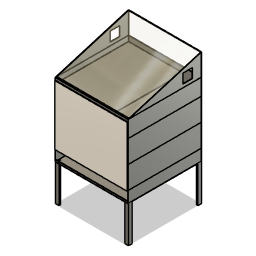
Solar Dryer Assembly v2 (Autodesk Fusion 360 archive; units mm, degrees)
design "Chamber Solar Dryer"
Autodesk Fusion 360 part; units mm, degrees
sketch "Sketch1" plane through (0, 0, 0) normal (0, 1, 0) x (1, 0, 0)
  line L0 (1000, 0) -> (1000, 1000)
  line L1 (1000, 1000) -> (0, 1000)
  line L2 (0, 1000) -> (0, 0)
  line L3 (996, 4) -> (996, 996)
  line L4 (996, 996) -> (4, 996)
  line L5 (4, 996) -> (4, 4)
  line L6 (996, 4) -> (996, 0)
  line L7 (996, 0) -> (1000, 0)
  line L8 (4, 4) -> (4, 0)
  line L9 (4, 0) -> (0, 0)
  dimension "d1" = 1000
  dimension "d2" = 1000
  dimension "d3" = 992
  dimension "d4" = 992
  constraint vertical L0
  constraint horizontal L1
  constraint vertical L2
  constraint coincident L2.end L9.end
  constraint vertical L3
  constraint horizontal L4
  constraint vertical L5
  constraint parallel L0 L6
  constraint perpendicular L0 L7
  constraint perpendicular L7 L8
  constraint perpendicular L2 L9
  measures "d1" distance of L2.end L0.start
  measures "d2" distance of L2.end L1.end
  measures "d3" distance of L5.end L3.start
  measures "d4" distance of L5.end L4.end
extrude "Extrude1" add sketch "Sketch1" along normal blind 1000 makes body 1
ref_plane "WorkPlane1" through (500, 500, -996) normal (0, 0, 1) x (1, 0, 0)
sketch "Sketch2" plane through (0, 0, -996) normal (0, 0, 1) x (1, 0, 0)
  line L0 (4, 0) -> (996, 0)
  line L1 (996, 0) -> (996, 4)
  line L2 (996, 4) -> (4, 4)
  line L3 (4, 4) -> (4, 0)
  dimension "d8" = 992
  dimension "d9" = 4
  constraint horizontal L0
  constraint vertical L1
  constraint horizontal L2
  constraint vertical L3
  measures "d8" distance of L0.start L0.end
  measures "d9" distance of L0.start L2.end
extrude "Extrude2" add sketch "Sketch2" along normal blind 996 bodies 1
ref_plane "WorkPlane2" through (500, 502, -996) normal (0, 0, 1) x (1, 0, 0)
sketch "Sketch3" plane through (0, 0, -996) normal (0, 0, 1) x (1, 0, 0)
  line L0 (4, 312) -> (4, 308)
  line L1 (996, 154) -> (246, 154)
  line L2 (246, 154) -> (246, 158)
  line L3 (246, 158) -> (996, 158)
  line L4 (996, 158) -> (996, 154)
  line L5 (754, 308) -> (754, 312)
  line L6 (754, 312) -> (4, 312)
  line L7 (246, 466) -> (996, 466)
  line L8 (246, 462) -> (246, 466)
  line L9 (996, 462) -> (246, 462)
  line L10 (4, 312) -> (4, 308)
  line L11 (4, 308) -> (754, 308)
  line L12 (996, 466) -> (996, 462)
  line L13 (754, 620) -> (4, 620)
  line L14 (996, 774) -> (996, 770)
  line L15 (246, 774) -> (996, 774)
  line L16 (4, 620) -> (4, 616)
  line L17 (4, 620) -> (4, 616)
  line L18 (996, 770) -> (246, 770)
  line L19 (4, 616) -> (754, 616)
  line L20 (754, 616) -> (754, 620)
  line L21 (246, 770) -> (246, 774)
  line L22 (754, 928) -> (4, 928)
  line L23 (754, 924) -> (754, 928)
  line L24 (4, 924) -> (754, 924)
  line L25 (4, 928) -> (4, 924)
  line L26 (4, 928) -> (4, 924)
  dimension "d14" = 4
  dimension "d15" = 750
  dimension "d16" = 4
  dimension "d17" = 750
  dimension "d18" = 4
  dimension "d19" = 750
  dimension "d20" = 4
  dimension "d21" = 750
  dimension "d22" = 4
  dimension "d24" = 4
  dimension "d25" = 750
  dimension "d26" = 4
  dimension "d27" = 750
  dimension "d28" = 4
  dimension "d30" = 4
  constraint vertical L0
  constraint horizontal L1
  constraint vertical L2
  constraint horizontal L3
  constraint vertical L4
  constraint horizontal L11
  constraint vertical L5
  constraint horizontal L6
  constraint vertical L10
  constraint horizontal L9
  constraint vertical L8
  constraint horizontal L7
  constraint vertical L12
  constraint horizontal L19
  constraint vertical L20
  constraint horizontal L13
  constraint vertical L17
  constraint vertical L16
  constraint horizontal L18
  constraint vertical L21
  constraint horizontal L15
  constraint vertical L14
  constraint horizontal L24
  constraint vertical L23
  constraint horizontal L22
  constraint vertical L26
  constraint vertical L25
  measures "d14" distance of L0.end L0.start
  measures "d15" distance of L1.start L1.end
  measures "d16" distance of L1.start L3.end
  measures "d17" distance of L0.end L5.start
  measures "d18" distance of L0.end L0.start
  measures "d19" distance of L9.start L8.start
  measures "d20" distance of L9.start L7.end
  measures "d21" distance of L16.end L19.end
  measures "d22" distance of L16.end L13.end
  measures "d24" distance of L13.end L16.end
  measures "d25" distance of L18.end L14.end
  measures "d26" distance of L14.end L14.start
  measures "d27" distance of L24.start L23.start
  measures "d28" distance of L24.start L22.end
  measures "d30" distance of L22.end L24.start
extrude "Extrude3" add sketch "Sketch3" along normal blind 992 separate body makes body 2 at (496, 466, -665.3333) makes body 3 at (746, 770, -665.3333) makes body 4 at (504, 312, -665.3333) makes body 5 at (254, 616, -665.3333) makes body 6 at (254, 924, -665.3333) makes body 7 at (746, 154, -665.3333)
ref_plane "WorkPlane3" through (4, 502, -498) normal (1, 0, 0) x (0, 0, -1)
sketch "Sketch4" plane through (4, 0, 0) normal (1, 0, 0) x (0, 0, -1)
  line L0 (1000, 1000) -> (1000, 1300)
  line L1 (1000, 1300) -> (0, 1000)
  line L2 (1000, 1000) -> (996, 1000)
  line L3 (0, 1000) -> (4, 1000)
  line L4 (996, 1000) -> (996, 1293)
  line L5 (996, 1293) -> (996, 1294)
  line L6 (996, 1294) -> (15.9999, 1000)
  line L7 (15.9999, 1000) -> (4, 1000)
  dimension "d34" = 300
  dimension "d35" = 4
  dimension "d36" = 4
  constraint vertical L0
  constraint perpendicular L0 L2
  constraint horizontal L3
  constraint perpendicular L2 L4
  constraint parallel L4 L5
  constraint parallel L1 L6
  constraint parallel L3 L7
  measures "d34" distance of L0.start L0.end
  measures "d35" distance of L0.start L2.end
  measures "d36" distance of L1.end L3.end
extrude "Extrude4" add sketch "Sketch4" along normal blind 992 separate body makes body 8
ref_plane "WorkPlane4" through (379, 926, -4) normal (0, 0, 1) x (1, 0, 0)
sketch "Sketch5" plane through (0, 0, -4) normal (0, 0, 1) x (1, 0, 0)
  line L0 (4, 305) -> (4, 315)
  line L1 (996, 161) -> (246, 161)
  line L2 (246, 161) -> (246, 151)
  line L3 (246, 151) -> (996, 151)
  line L4 (996, 151) -> (996, 161)
  line L5 (996, 767) -> (996, 777)
  line L6 (246, 767) -> (996, 767)
  line L7 (996, 777) -> (246, 777)
  line L8 (246, 777) -> (246, 767)
  line L9 (4, 931) -> (754, 931)
  line L10 (754, 921) -> (4, 921)
  line L11 (4, 921) -> (4, 931)
  line L12 (754, 931) -> (754, 921)
  line L13 (996, 469) -> (246, 469)
  line L14 (996, 459) -> (996, 469)
  line L15 (754, 315) -> (754, 305)
  line L16 (754, 305) -> (4, 305)
  line L17 (4, 315) -> (754, 315)
  line L18 (246, 459) -> (996, 459)
  line L19 (246, 469) -> (246, 459)
  line L20 (4, 305) -> (4, 315)
  line L21 (4, 613) -> (754, 613)
  line L22 (754, 613) -> (754, 623)
  line L23 (754, 623) -> (4, 623)
  line L24 (4, 623) -> (4, 613)
  dimension "d41" = 10
  dimension "d42" = 750
  dimension "d43" = 10
  dimension "d44" = 750
  dimension "d45" = 10
  dimension "d46" = 750
  dimension "d47" = 10
  dimension "d48" = 750
  dimension "d49" = 10
  dimension "d50" = 750
  dimension "d51" = 10
  dimension "d52" = 750
  dimension "d53" = 10
  constraint vertical L0
  constraint horizontal L1
  constraint vertical L2
  constraint horizontal L3
  constraint vertical L4
  constraint horizontal L7
  constraint vertical L8
  constraint horizontal L6
  constraint vertical L5
  constraint horizontal L9
  constraint vertical L12
  constraint horizontal L10
  constraint vertical L11
  constraint horizontal L17
  constraint vertical L15
  constraint horizontal L16
  constraint vertical L20
  constraint horizontal L13
  constraint vertical L19
  constraint horizontal L18
  constraint vertical L14
  constraint horizontal L21
  constraint vertical L22
  constraint horizontal L23
  constraint vertical L24
  measures "d41" distance of L0.end L0.start
  measures "d42" distance of L1.start L1.end
  measures "d43" distance of L1.start L3.end
  measures "d44" distance of L5.end L7.end
  measures "d45" distance of L5.end L5.start
  measures "d46" distance of L9.start L9.end
  measures "d47" distance of L10.end L9.start
  measures "d48" distance of L0.end L15.start
  measures "d49" distance of L0.start L0.end
  measures "d50" distance of L13.start L13.end
  measures "d51" distance of L13.start L14.start
  measures "d52" distance of L21.start L21.end
  measures "d53" distance of L21.start L23.end
extrude "Extrude5" add sketch "Sketch5" along normal blind 4 bodies 1 2 3 4 5 6 7
ref_plane "WorkPlane5" through (996, 1150, -500) normal (1, 0, 0) x (0, 0, -1)
sketch "Sketch6" plane through (996, 0, 0) normal (1, 0, 0) x (0, 0, -1)
  line L0 (875, 1175) -> (745, 1175)
  line L1 (745, 1175) -> (745, 1045)
  line L2 (745, 1045) -> (875, 1045)
  line L3 (875, 1045) -> (875, 1175)
  line L4 (1000, 1000) -> (1000, 1300)
  line L5 (1000, 1300) -> (0, 1000)
  line L6 (0, 1000) -> (1000, 1000)
  dimension "d57" = 130
  dimension "d58" = 130
  constraint horizontal L0
  constraint vertical L1
  constraint horizontal L2
  constraint vertical L3
  constraint parallel L3 L4
  constraint perpendicular L4 L6
  measures "d57" distance of L0.start L0.end
  measures "d58" distance of L0.start L2.end
extrude "Extrude6" add sketch "Sketch6" along normal blind 4 separate body makes body 9
sketch "Sketch7" plane through (4, 0, 0) normal (-1, 0, 0) x (0, 0, 1)
  line L0 (-1000, 1300) -> (-1000, 1000)
  line L1 (-1000, 1000) -> (-996, 1000)
  line L2 (-996, 1000) -> (-996, 1294)
  line L3 (-996, 1294) -> (-15.9999, 1000)
  line L4 (-15.9999, 1000) -> (0, 1000)
  line L5 (0, 1000) -> (-1000, 1300)
  line L6 (-1000, 1300) -> (-1000, 1000)
  line L7 (-1000, 1300) -> (0, 1000)
  line L8 (0, 1000) -> (-1000, 1000)
  line L9 (-875, 1175) -> (-745, 1175)
  line L10 (-745, 1175) -> (-745, 1045)
  line L11 (-745, 1045) -> (-875, 1045)
  line L12 (-875, 1045) -> (-875, 1175)
  constraint coincident L0.start L5.end
  constraint coincident L0.end L1.start
  constraint coincident L4.end L5.start
  constraint horizontal L9
  constraint vertical L10
  constraint horizontal L11
  constraint vertical L12
extrude "Extrude7" add sketch "Sketch7" along normal blind 4 separate body makes body 10
ref_plane "WorkPlane6" through (500, 500, 0) normal (0, 0, 1) x (1, 0, 0)
sketch "Sketch8" plane through (0, 0, 0) normal (0, 0, 1) x (1, 0, 0)
  line L0 (0, 0) -> (1000, 0)
  line L1 (1000, 0) -> (1000, 1000)
  line L2 (1000, 1000) -> (0, 1000)
  line L3 (0, 1000) -> (0, 0)
  line L4 (4, 25.0504) -> (996, 25.0504)
  line L5 (996, 25.0504) -> (996, 968)
  line L6 (996, 968) -> (4, 968)
  line L7 (4, 968) -> (4, 25.0504)
  constraint horizontal L0
  constraint vertical L1
  constraint horizontal L2
  constraint vertical L3
  constraint coincident L0.start L3.end
  constraint horizontal L4
  constraint vertical L5
  constraint horizontal L6
  constraint vertical L7
extrude "Extrude8" add sketch "Sketch8" along normal blind 6 separate body makes body 11
ref_plane "WorkPlane7" through (500, 500, 6) normal (0, 0, 1) x (1, 0, 0)
sketch "Sketch9" plane through (0, 0, 6) normal (0, 0, 1) x (1, 0, 0)
  line L0 (4, 150.5002) -> (996, 150.5002)
  line L1 (996, 150.5002) -> (996, 968)
  line L2 (996, 968) -> (4, 968)
  line L3 (4, 968) -> (4, 150.5002)
  constraint horizontal L0
  constraint vertical L1
  constraint horizontal L2
  constraint vertical L3
extrude "Extrude9" add sketch "Sketch9" along normal blind 8 separate body makes body 12
ref_plane "WorkPlane8" through (500, 0, -500) normal (0, -1, 0) x (-1, 0, 0)
sketch "Sketch10" plane through (0, 0, 0) normal (0, -1, 0) x (-1, 0, 0)
  line L0 (0, 0) -> (0, 50)
  line L1 (0, 50) -> (-20, 50)
  line L2 (0, 0) -> (-50, 0)
  line L3 (-50, 0) -> (-50, 20)
  line L4 (-50, 20) -> (-20, 20)
  line L5 (-20, 20) -> (-20, 35)
  line L6 (-1000, 0) -> (-950, 0)
  line L7 (-950, 0) -> (-950, 20)
  line L8 (-1000, 0) -> (-1000, 50)
  line L9 (-1000, 50) -> (-980, 50)
  line L10 (-950, 20) -> (-980, 20)
  line L11 (-980, 20) -> (-980, 50)
  line L12 (-1000, 1000) -> (-1000, 950)
  line L13 (-1000, 950) -> (-980, 950)
  line L14 (-1000, 1000) -> (-950, 1000)
  line L15 (-950, 1000) -> (-950, 980)
  line L16 (-950, 980) -> (-980, 980)
  line L17 (-980, 980) -> (-980, 950)
  line L18 (0, 1000) -> (0, 950)
  line L19 (0, 950) -> (-20, 950)
  line L20 (0, 1000) -> (-50, 1000)
  line L21 (-50, 1000) -> (-50, 980)
  line L22 (-50, 980) -> (-20, 980)
  line L23 (-20, 980) -> (-20, 950)
  line L24 (-20, 35) -> (-20, 50)
  dimension "d70" = 50
  dimension "d71" = 20
  dimension "d72" = 50
  dimension "d73" = 20
  dimension "d74" = 50
  dimension "d75" = 20
  dimension "d76" = 50
  dimension "d77" = 20
  dimension "d78" = 50
  dimension "d79" = 50
  dimension "d80" = 20
  constraint coincident L0.start L2.start
  constraint vertical L0
  constraint perpendicular L0 L1
  constraint perpendicular L0 L2
  constraint perpendicular L2 L3
  constraint perpendicular L3 L4
  constraint perpendicular L4 L5
  constraint horizontal L6
  constraint perpendicular L6 L7
  constraint perpendicular L6 L8
  constraint perpendicular L8 L9
  constraint perpendicular L7 L10
  constraint perpendicular L9 L11
  constraint vertical L12
  constraint perpendicular L12 L13
  constraint perpendicular L12 L14
  constraint perpendicular L14 L15
  constraint perpendicular L15 L16
  constraint perpendicular L13 L17
  constraint perpendicular L14 L18
  constraint perpendicular L17 L19
  constraint perpendicular L18 L20
  constraint perpendicular L20 L21
  constraint perpendicular L21 L22
  constraint perpendicular L19 L23
  constraint perpendicular L1 L24
  measures "d70" distance of L0.start L0.end
  measures "d71" distance of L0.end L1.end
  measures "d72" distance of L0.start L2.end
  measures "d73" distance of L2.end L3.end
  measures "d74" distance of L6.start L6.end
  measures "d75" distance of L6.end L7.end
  measures "d76" distance of L6.start L8.end
  measures "d77" distance of L8.end L9.end
  measures "d78" distance of L12.start L12.end
  measures "d79" distance of L12.start L14.end
  measures "d80" distance of L14.end L15.end
extrude "Extrude10" add sketch "Sketch10" along normal blind 500 bodies 1 12 11

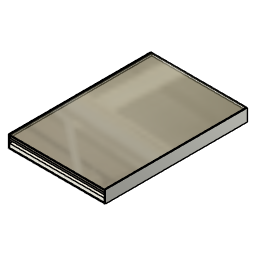
design "Solar Collector"
Autodesk Fusion 360 part; units mm, degrees
sketch "Sketch1" plane through (0, 0, 0) normal (0, 0, 1) x (1, 0, 0)
  line L0 (0, 0) -> (1000, 0)
  line L1 (1000, 0) -> (1000, 40)
  line L2 (1000, 40) -> (0, 40)
  line L3 (0, 40) -> (0, 0)
  line L4 (0, 90) -> (1000, 90)
  line L5 (1000, 90) -> (1000, 70)
  line L6 (1000, 70) -> (0, 70)
  line L7 (0, 70) -> (0, 90)
  line L8 (0, 120) -> (1000, 120)
  line L9 (1000, 120) -> (1000, 110)
  line L10 (1000, 110) -> (0, 110)
  line L11 (0, 110) -> (0, 120)
  line L12 (0, 120) -> (-10, 120)
  line L13 (-10, 120) -> (-10, -10)
  line L14 (-10, -10) -> (1000, -10)
  line L15 (1000, -10) -> (1010, -10)
  line L16 (1010, -10) -> (1010, 120)
  line L17 (1010, 120) -> (1000, 120)
  line L18 (1000, 0) -> (1000, 120)
  line L19 (0, 120) -> (0, 0)
  dimension "d1" = 1000
  dimension "d2" = 40
  dimension "d3" = 1000
  dimension "d4" = 20
  dimension "d5" = 1000
  dimension "d6" = 10
  dimension "d7" = 10
  dimension "d8" = 1010
  constraint horizontal L0
  constraint vertical L1
  constraint horizontal L2
  constraint vertical L3
  constraint coincident L0.start L3.end
  constraint horizontal L4
  constraint vertical L5
  constraint horizontal L6
  constraint vertical L7
  constraint horizontal L8
  constraint vertical L9
  constraint horizontal L10
  constraint vertical L11
  constraint perpendicular L11 L12
  constraint perpendicular L8 L13
  constraint perpendicular L13 L14
  constraint perpendicular L1 L15
  constraint perpendicular L2 L16
  constraint parallel L9 L18
  measures "d1" distance of L0.start L0.end
  measures "d2" distance of L0.start L2.end
  measures "d3" distance of L4.start L4.end
  measures "d4" distance of L4.start L6.end
  measures "d5" distance of L8.start L8.end
  measures "d6" distance of L8.start L10.end
  measures "d7" distance of L8.start L12.end
  measures "d8" distance of L13.end L14.end
sketch "Sketch2" plane through (0, 0, 0) normal (0, 0, 1) x (1, 0, 0)
  line L0 (0, 0) -> (1000, 0)
  line L1 (1000, 0) -> (1000, 40)
  line L2 (1000, 40) -> (0, 40)
  line L3 (0, 40) -> (0, 0)
  dimension "d11" = 1000
  dimension "d12" = 40
  constraint horizontal L0
  constraint vertical L1
  constraint horizontal L2
  constraint vertical L3
  constraint coincident L0.start L3.end
  measures "d11" distance of L0.start L0.end
  measures "d12" distance of L0.start L2.end
sketch "Sketch3" plane through (0, 0, 0) normal (0, 0, 1) x (1, 0, 0)
  line L0 (0, 70) -> (1000, 70)
  line L1 (1000, 70) -> (1000, 90)
  line L2 (1000, 90) -> (0, 90)
  line L3 (0, 90) -> (0, 70)
  dimension "d15" = 1000
  dimension "d16" = 20
  constraint horizontal L0
  constraint vertical L1
  constraint horizontal L2
  constraint vertical L3
  measures "d15" distance of L0.start L0.end
  measures "d16" distance of L0.start L2.end
sketch "Sketch4" plane through (0, 0, 1400) normal (0, 0, 1) x (1, 0, 0)
  line L0 (0, 40) -> (0, 0)
  line L1 (0, 0) -> (1000, 0)
  line L2 (1000, 0) -> (1000, 40)
  line L3 (1000, 40) -> (0, 40)
  line L4 (0, 120) -> (1000, 120)
  line L5 (1000, 120) -> (1000, 110)
  line L6 (1000, 110) -> (0, 110)
  line L7 (0, 110) -> (0, 120)
  dimension "d19" = 1000
  dimension "d20" = 10
  constraint horizontal L4
  constraint vertical L5
  constraint horizontal L6
  constraint vertical L7
  measures "d19" distance of L4.start L4.end
  measures "d20" distance of L4.start L6.end
extrude "Extrude5" add sketch "Sketch1" along normal blind 1500 contours L0 L1 L3 L5 L7 L9 L11 L12 L13 L14 L15 L16 L17 L18 L19 makes body 1
extrude "Extrude6" add sketch "Sketch2" along normal blind 1500 separate body makes body 2
extrude "Extrude7" add sketch "Sketch3" along normal blind 1500 separate body makes body 3
extrude "Extrude8" add sketch "Sketch4" along normal blind 100 and the other way blind 1400 separate body contours L4 L5 L6 L7 makes body 4
